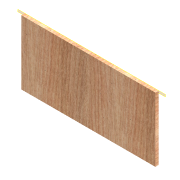
# Autodesk Inventor part: boevenkant doos
Saved by Autodesk Inventor 2020.3 (Build 243373000, 373)
## iProperties
Created: 2020-10-19
Part Number: boevenkant doos
Material: Wood (Birch)
Document SubType Name: Sheet Metal
Designer: Svend
Density: 0.55 g/cm^3
Sheet Metal Rule: Default_mm
Appearance: Birch - Natural Polished
Author: Svend
Autodesk Inventor part; units mm, degrees
ref_plane "YZ Plane" through (0, 0, 0) normal (1, 0, 0) x (0, 1, 0)
ref_plane "XZ Plane" through (0, 0, 0) normal (0, 1, 0) x (-1, 0, 0)
ref_plane "XY Plane" through (0, 0, 0) normal (0, 0, 1) x (1, 0, 0)
ref_plane "Work Plane1" through (0, 0, 0) normal (0, 0, 1) x (1, 0, 0)
sketch "Sketch1" plane through (0, 0, 0) normal (0, 0, 1) x (1, 0, 0)
  line L0 (0, 6) -> (-400, 6) projected
  line L1 (-400, 0) -> (-400, 6) projected
  line L2 (-400, 0) -> (0, 0) projected
  line L3 (0, 0) -> (0, 6) projected
  line L4 (-6, 0) -> (-6, -179.7467) projected
  line L5 (0, -179.7467) -> (-6, -179.7467) projected
  line L6 (0, -179.7467) -> (0, 0) projected
  line L7 (0, 0) -> (-6, 0) projected
  line L8 (0, -179.7467) -> (-400, -179.7467) projected
  line L9 (-400, -185.7467) -> (-400, -179.7467) projected
  line L10 (-400, -185.7467) -> (0, -185.7467) projected
  line L11 (0, -185.7467) -> (0, -179.7467) projected
  line L12 (-394, -179.7467) -> (-394, 0) projected
  line L13 (-400, 0) -> (-394, 0) projected
  line L14 (-400, 0) -> (-400, -179.7467) projected
  line L15 (-400, -179.7467) -> (-394, -179.7467) projected
  line L16 (-400, 6) -> (0, 6)
  line L17 (0, 6) -> (0, -185.7467)
  line L18 (0, -185.7467) -> (-400, -185.7467)
  line L19 (-400, -185.7467) -> (-400, 6)
  constraints: 8 end point, 2 parallel, 1 horizontal, 1 perpendicular
extrude "Extrusion1" add sketch "Sketch1" along normal blind 10
equation "\"BendRadius\" = Thickness"
equation "\"BendReliefWidth\" = Thickness"
equation "\"BendReliefDepth\" = 0.5 * Thickness"
equation "\"CornerReliefSize\" = 4 * Thickness"
equation "\"MinimumRemnant\" = 2 * Thickness"
equation "\"TransitionRadius\" = BendRadius"
equation "\"JacobiRadiusSize\" = BendRadius"
equation "\"GapSize\" = Thickness"
equation "\"Thickness\" = 6"
body "Solid1"
